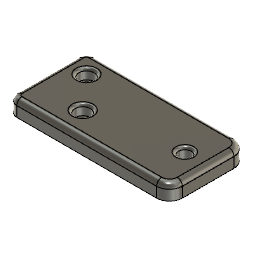
pfte_halter_2 (Autodesk Fusion 360 design; units mm, degrees)
part number: 2026-03-28-21-58-07-381
Autodesk Fusion 360 part; units mm, degrees
sketch "Sketch1" plane through (0, 0, 0) normal (0, 0, 1) x (1, 0, 0)
  circle A0 centre (0, 0) radius 2
  circle A1 centre (11.2624, -12.7341) radius 2
  circle A2 centre (11.2624, -12.7341) radius 3
  circle A3 centre (0, 0) radius 3
  line L0 (-8, 8) -> (54, 8)
  line L1 (54, 8) -> (54, -21.9327)
  line L2 (54, -21.9327) -> (-8, -21.9327)
  line L3 (-8, -21.9327) -> (-8, 8)
  circle A4 centre (45, -7) radius 2.5
  dimension "d1" = 4
  dimension "d2" = 4
  dimension "d3" = 6
  dimension "d4" = 6
  dimension "d5" = 17
  dimension "d6" = 5
  constraint coincident A0.centre A3.centre
  constraint concentric A1 A2
  constraint concentric A0 A3
  constraint horizontal L0
  constraint vertical L1
  constraint horizontal L2
  constraint vertical L3
  measures "d1" diameter of A0
  measures "d2" diameter of A1
  measures "d3" diameter of A2
  measures "d4" diameter of A3
  measures "d5" distance of A1.centre A0.centre
  measures "d6" diameter of A4
extrude "Extrude1" add sketch "Sketch1" against normal blind 6 contours A2 | A3 | L0 L1 L2 L3
extrude "Extrude2" cut sketch "Sketch1" against normal blind 4 contours A2 | A3
fillet "Fillet1" radius 5 2 edges at (54, -21.9327, -3) (54, 8, -3)
fillet "Fillet2" radius 3 2 edges at (-8, -21.9327, -3) (-8, 8, -3)
fillet "Fillet3" radius 2 8 edges at (-8, -6.9663, 0) (-7.1213, 7.1213, 0) (22, 8, 0) (52.5355, 6.5355, 0) (54, -6.9663, 0) (52.5355, -20.4682, 0) (22, -21.9327, 0) (-7.1213, -21.054, 0)
fillet "Fillet4" radius 1 3 edges at (42.6692, -6.096, 0) (8.4654, -11.6493, 0) (-2.797, 1.0848, 0)
